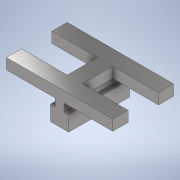
# Autodesk Inventor part: barrier_pneumatic_connector
Saved by Autodesk Inventor 2022 (Build 260153000, 153)
## iProperties
Created: 2021-11-08
Part Number: barrier_pneumatic_connector
Material: Stainless Steel
Document SubType Name: Modeling
Designer: kibandi
Density: 8 g/cm^3
Appearance: Semi-Polished
Mass: 137600 g
Surface Area: 7560 cm^2
Volume: 17200 cm^3
Author: kibandi
Autodesk Inventor part; units mm, degrees
ref_plane "YZ Plane" through (0, 0, 0) normal (1, 0, 0) x (0, 1, 0)
ref_plane "XZ Plane" through (0, 0, 0) normal (0, 1, 0) x (-1, 0, 0)
ref_plane "XY Plane" through (0, 0, 0) normal (0, 0, 1) x (1, 0, 0)
sketch "Sketch1" plane through (0, 0, 0) normal (0, 1, 0) x (-1, 0, 0)
  line L0 (0, 0) -> (700, 0)
  line L1 (700, 0) -> (700, -100)
  line L2 (700, -100) -> (400, -100)
  line L3 (400, -100) -> (400, -300)
  line L4 (400, -300) -> (700, -300)
  line L5 (700, -300) -> (700, -400)
  line L6 (700, -400) -> (0, -400)
  line L7 (0, -400) -> (0, -300)
  line L8 (0, -300) -> (300, -300)
  line L9 (300, -300) -> (300, -100)
  line L10 (300, -100) -> (0, -100)
  line L11 (0, -100) -> (0, 0)
  dimension "d0" = 700
  dimension "d1" = 100
  dimension "d2" = 300
  dimension "d3" = 200
  dimension "d4" = 100
  dimension "d5" = 700
  dimension "d6" = 300
  constraints: 24 end point, 7 perpendicular, 7 point on line, 1 horizontal
  measures "d0" distance of L0.start L0.end
  measures "d1" distance of L0.end L1.end
  measures "d2" distance of L1.end L2.end
  measures "d3" distance of L2.end L3.end
  measures "d4" distance of L4.end L5.end
  measures "d5" distance of L5.end L6.end
  measures "d6" distance of L7.end L8.end
extrude "Extrusion1" add sketch "Sketch1" along normal blind 70
sketch "Sketch2" plane through (-700, 0, 0) normal (0, 0, 1) x (1, 0, 0)
  line L0 (700, 0) -> (0, 0) projected
  line L1 (350, 0) -> (380, 0)
  line L2 (380, 0) -> (320, 0)
  line L3 (320, 0) -> (320, -50)
  line L4 (320, -50) -> (290, -50)
  line L5 (290, -50) -> (290, -150)
  line L6 (290, -150) -> (410, -150)
  line L7 (410, -150) -> (410, -50)
  line L8 (410, -50) -> (380, -50)
  line L9 (380, -50) -> (380, 0)
  dimension "d9" = 30
  dimension "d10" = 60
  dimension "d11" = 50
  dimension "d12" = 30
  dimension "d13" = 100
  dimension "d14" = 120
  dimension "d15" = 30
  constraints: 18 end point, 4 perpendicular, 4 point on line, 1 horizontal, 1 midpoint
  measures "d9" distance of L1.start L1.end
  measures "d10" distance of L1.end L2.end
  measures "d11" distance of L2.end L3.end
  measures "d12" distance of L3.end L4.end
  measures "d13" distance of L4.end L5.end
  measures "d14" distance of L5.end L6.end
  measures "d15" distance of L7.end L8.end
extrude "Extrusion2" add sketch "Sketch2" against normal blind 400
body "Solid1"
